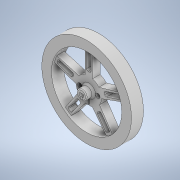
# Autodesk Inventor part: Колесо D60 под ось моторов серии N
Saved by Autodesk Inventor 2020 (Build 240168000, 168)
## iProperties
Created: 2021-03-21
Part Number: Колесо D60 под ось моторов серии N
Material: Типовые
Document SubType Name: Modeling
Designer: Антон
Density: 1 g/cm^3
Appearance: По умолчанию
Author: Антон
Autodesk Inventor part; units mm, degrees
ref_plane "YZ Plane" through (0, 0, 0) normal (1, 0, 0) x (0, 1, 0)
ref_plane "XZ Plane" through (0, 0, 0) normal (0, 1, 0) x (-1, 0, 0)
ref_plane "XY Plane" through (0, 0, 0) normal (0, 0, 1) x (1, 0, 0)
sketch "Эскиз1" plane through (0, 0, 0) normal (0, 0, 1) x (1, 0, 0)
  circle A0 centre (0, 0) radius 30
  circle A1 centre (0, 0) radius 23.5
  dimension "d0" = 60
  dimension "d1" = 47
  constraints: 2 centre point, 2 coincident
  measures "d0" diameter of A0
  measures "d1" diameter of A1
extrude "Выдавливание1" add sketch "Эскиз1" along normal blind 8
ref_plane "РабПлоскость1" through (0, 0, 4) normal (0, 0, 1) x (1, 0, 0)
sketch "Эскиз2" plane through (0, 0, 4) normal (0, 0, 1) x (1, 0, 0)
  circle A0 centre (0, 0) radius 8.5
  line L0 (3, -23.5) -> (3, 23.5)
  line L1 (3, 23.5) -> (-3, 23.5)
  line L2 (-3, 23.5) -> (-3, -23.5)
  line L3 (-3, -23.5) -> (3, -23.5)
  line L4 (3, -23.5) -> (-3, 23.5) construction
  line L5 (3, 23.5) -> (-3, -23.5) construction
  line L6 (2.5, -23.5) -> (2.5, 23.5)
  line L7 (2.5, 23.5) -> (-2.5, 23.5)
  line L8 (-2.5, 23.5) -> (-2.5, -23.5)
  line L9 (-2.5, -23.5) -> (2.5, -23.5)
  line L10 (2.5, -23.5) -> (-2.5, 23.5) construction
  line L11 (2.5, 23.5) -> (-2.5, -23.5) construction
  circle A1 centre (0, 0) radius 23.5 projected
  line L12 (-2.486, 23.3681) -> (-3, 7.953)
  line L13 (2.486, 23.3681) -> (3, 7.953)
  circle A2 centre (0, 0) radius 1.5
  line L14 (-1.5, -1) -> (1.5, -1)
  line L15 (1.5, -1) -> (1.5, 1)
  line L16 (1.5, 1) -> (-1.5, 1)
  line L17 (-1.5, 1) -> (-1.5, -1)
  line L18 (-1.5, -1) -> (1.5, 1) construction
  line L19 (1.5, -1) -> (-1.5, 1) construction
  line L20 (0, 0) -> (0, -8.5)
  line L21 (0.5, -8.5) -> (0.5, 0)
  line L22 (0.5, 0) -> (-0.5, 0)
  line L23 (-0.5, 0) -> (-0.5, -8.5)
  line L24 (-0.5, -8.5) -> (0.5, -8.5)
  line L25 (0.5, -8.5) -> (-0.5, 0) construction
  line L26 (0.5, 0) -> (-0.5, -8.5) construction
  line L27 (0, 0) -> (6, 0)
  line L28 (0, 0) -> (-6, 0)
  circle A3 centre (-6, 0) radius 1.5
  circle A4 centre (6, 0) radius 1.5
  line L29 (0, 0) -> (0, 16.5)
  line L30 (-1.5, 11) -> (1.5, 11)
  line L31 (1.5, 11) -> (1.5, 22)
  line L32 (1.5, 22) -> (-1.5, 22)
  line L33 (-1.5, 22) -> (-1.5, 11)
  line L34 (-1.5, 11) -> (1.5, 22) construction
  line L35 (1.5, 11) -> (-1.5, 22) construction
  line L36 (-22.9926, 4.8569) -> (-8.4908, -0.3956)
  circle A5 centre (0, 0) radius 8.5
  line L37 (-21.4562, 9.5855) -> (-6.6367, 5.3108)
  line L38 (-21.3868, 5.3718) -> (-10.9251, 1.9726)
  line L39 (-20.4597, 8.225) -> (-21.3868, 5.3718)
  line L40 (-9.9981, 4.8258) -> (-20.4597, 8.225)
  line L41 (-10.9251, 1.9726) -> (-9.9981, 4.8258)
  line L42 (-21.4228, 10.1151) -> (-23.2769, 4.4087)
  line L43 (-11.7243, -20.3664) -> (-2.2476, -8.1975)
  circle A6 centre (0, 0) radius 8.5
  line L44 (-15.7466, -17.444) -> (-7.1017, -4.6707)
  line L45 (-11.7178, -18.6801) -> (-5.2521, -9.7809)
  line L46 (-14.1448, -16.9167) -> (-11.7178, -18.6801)
  line L47 (-7.6792, -8.0175) -> (-14.1448, -16.9167)
  line L48 (-5.2521, -9.7809) -> (-7.6792, -8.0175)
  line L49 (-16.24, -17.2485) -> (-11.3859, -20.7753)
  line L50 (15.7466, -17.444) -> (7.1017, -4.6707)
  circle A7 centre (0, 0) radius 8.5
  line L51 (11.7243, -20.3664) -> (2.2476, -8.1975)
  line L52 (14.1448, -16.9167) -> (7.6792, -8.0175)
  line L53 (11.7178, -18.6801) -> (14.1448, -16.9167)
  line L54 (5.2521, -9.7809) -> (11.7178, -18.6801)
  line L55 (7.6792, -8.0175) -> (5.2521, -9.7809)
  line L56 (11.3859, -20.7753) -> (16.24, -17.2485)
  line L57 (21.4562, 9.5855) -> (6.6367, 5.3108)
  circle A8 centre (0, 0) radius 8.5
  line L58 (22.9926, 4.8569) -> (8.4908, -0.3956)
  line L59 (20.4597, 8.225) -> (9.9981, 4.8258)
  line L60 (21.3868, 5.3718) -> (20.4597, 8.225)
  line L61 (10.9251, 1.9726) -> (21.3868, 5.3718)
  line L62 (9.9981, 4.8258) -> (10.9251, 1.9726)
  line L63 (23.2769, 4.4087) -> (21.4228, 10.1151)
  point P0 (0, -4.25)
  point P1 (-0.5, -8.4853)
  point P2 (-0.5, -1.4142)
  point P3 (-1.118, 1)
  point P4 (1.118, 1)
  point P5 (0.5, -1.4142)
  point P6 (0.5, -8.4853)
  point P7 (2.5, 8.124)
  point P8 (2.5, 22.9475)
  point P9 (-2.5, 22.9475)
  point P10 (-2.5, 8.124)
  point P11 (-2.2476, -8.1975)
  point P12 (6.6367, 5.3108)
  dimension "d4" = 17
  dimension "d5" = 6
  dimension "d6" = 5
  dimension "d17" = 3
  dimension "d18" = 2
  dimension "d19" = 1
  dimension "d20" = 6
  dimension "d21" = 6
  dimension "d22" = 3
  dimension "d23" = 3
  dimension "d24" = 16.5
  dimension "d25" = 3
  dimension "d26" = 11
  dimension "d29" = 360
  constraints: 128 end point, 12 point on circle, 11 midpoint, 11 parallel, 8 centre point, 5 perpendicular, 4 horizontal, 4 point on line, 3 coincident, 3 vertical, 96 other
  measures "d4" diameter of A0
  measures "d5" distance of L1.end L0.end
  measures "d6" distance of L7.end L6.end
  measures "d17" diameter of A2
  measures "d18" distance of L15.end L14.end
  measures "d19" distance of L22.end L21.end
  measures "d20" distance of L20.start L27.end
  measures "d21" distance of L20.start L28.end
  measures "d22" diameter of A3
  measures "d23" diameter of A4
  measures "d24" distance of L20.start L29.end
  measures "d25" distance of L32.end L31.end
  measures "d26" distance of L31.end L30.end
extrude "Выдавливание2" add sketch "Эскиз2" along normal mid plane 5 contours A0 L0 | A0 L57 A1 L58 | L0 L27 L6 A0 | L50 A1 L51 L0 A0 | L6 L27 L15 L16 A2 L29 A0 | A0 L8 L12 A1 L13 L6 | L0 A0 L6 L27 | L0 L51 L6 A0 | L29 A2 L16 L17 L28 L8 A0 | L6 A0 L21 A2 L14 L15 L27 | L6 L51 A0 | L8 L28 L2 A0 | L29 L16 A2 | A2 L16 L29 | L15 L14 A2 | A2 L16 L15 | L2 A0 | L28 L17 L14 A2 L23 A0 L8 | L8 A0 L2 L28 | A2 L17 L16 | A0 L36 A1 L37 | L8 L43 L2 A0 | A0 L43 L8 | A2 L14 L17 | L2 L43 A1 L44 A0
fillet "Сопряжение1" radius 1 10 edges at (-9.9981, 4.8258, 4) (-10.9251, 1.9726, 4) (-7.6792, -8.0175, 4) (-5.2521, -9.7809, 4) (-1.5, 11, 4) (1.5, 11, 4) (5.2521, -9.7809, 4) (7.6792, -8.0175, 4) (10.9251, 1.9726, 4) (9.9981, 4.8258, 4)
fillet "Сопряжение2" radius 0.5 10 edges at (-14.1448, -16.9167, 4) (-11.7178, -18.6801, 4) (-20.4597, 8.225, 4) (-21.3868, 5.3718, 4) (1.5, 22, 4) (-1.5, 22, 4) (20.4597, 8.225, 4) (21.3868, 5.3718, 4) (14.1448, -16.9167, 4) (11.7178, -18.6801, 4)
sketch "Эскиз4" plane through (0, 0, 6.5) normal (0, 0, 1) x (1, 0, 0)
  circle A0 centre (0, 0) radius 3.25
  line L0 (-0.5, -8.4853) -> (-0.5, -1.4142) projected
  line L1 (0.5, -1.4142) -> (0.5, -8.4853) projected
  arc A1 (0.5, -1.4142) -> (1.118, 1) centre (0, 0) ccw projected
  arc A2 (-1.118, 1) -> (-0.5, -1.4142) centre (0, 0) ccw projected
  line L2 (-1.118, 1) -> (1.118, 1) projected
  point P0 (0.5, -3.2113)
  point P1 (-0.5, -3.2113)
  dimension "d34" = 6.5
  constraints: 1 centre point, 1 coincident
  measures "d34" diameter of A0
extrude "Выдавливание3" add sketch "Эскиз4" along normal blind 5 contours A0 L1 A1 L2 A2 L0 picked at (-0.1172, 1.7436)
fillet "Сопряжение3" radius 0.6 1 edges at (0, 3.25, 11.5)
fillet "Сопряжение4" radius 1.25 1 edges at (0, 3.25, 6.5)
